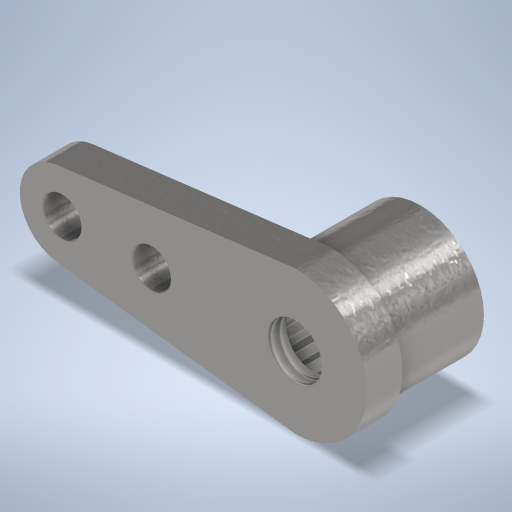
# Autodesk Inventor part: ara parca2
Saved by Autodesk Inventor 2023 (Build 270158000, 158)
## iProperties
Created: 2023-02-02
Part Number: ara parca2
Material: Generic
Document SubType Name: Sheet Metal
Designer: omuru
Density: 1 g/cm^3
Sheet Metal Rule: Default_mm
Appearance: Default
Author: omuru
Autodesk Inventor part; units mm, degrees
ref_plane "YZ Plane" through (0, 0, 0) normal (1, 0, 0) x (0, 1, 0)
ref_plane "XZ Plane" through (0, 0, 0) normal (0, 1, 0) x (-1, 0, 0)
ref_plane "XY Plane" through (0, 0, 0) normal (0, 0, 1) x (1, 0, 0)
sketch "Sketch1" plane through (0, 0, 0) normal (0, 0, 1) x (1, 0, 0)
  circle A0 centre (0, 0) radius 4
  circle A1 centre (0, 0) radius 3.5
  line L0 (0, 0) -> (-13, 0)
  line L1 (-13, 0) -> (-13, 0)
  circle A2 centre (-13, 0) radius 1.075
  line L2 (-13, 0) -> (-8, 0)
  circle A3 centre (-8, 0) radius 1.075
  arc A4 (-13.2917, 2.3513) -> (-13.2917, -2.3513) centre (-13, 0) ccw
  line L3 (0, 4) -> (-13.2917, 2.3513)
  line L4 (0, -4) -> (-13.2917, -2.3513)
  dimension "d0" = 8
  dimension "d1" = 7
  dimension "d5" = 2.15
  dimension "d7" = 2.15
  dimension "d31" = 8
  dimension "d33" = 5
  constraints: 10 end point, 6 coincident, 5 centre point, 4 point on circle, 2 point on line, 2 tangent, 1 horizontal
  measures "d0" diameter of A0
  measures "d1" diameter of A1
  measures "d5" diameter of A2
  measures "d7" diameter of A3
  measures "d31" distance of point (0, 0) L2.end
  measures "d33" distance of A3.centre L2.start
extrude "Extrusion1" add sketch "Sketch1" along normal mid plane 2 contours A0 L4 L3 | A0 L4 A4 L3
sketch "Sketch2" plane through (0, 0, -1) normal (0, 0, -1) x (-1, 0, 0)
  circle A0 centre (0, 0) radius 2.5
  circle A1 centre (0, 0) radius 4
  dimension "d11" = 5
  constraints: 2 centre point, 2 coincident
  measures "d11" diameter of A0
extrude "Extrusion2" add sketch "Sketch2" against normal blind 1
sketch "Sketch3" plane through (0, 0, 1) normal (0, 0, 1) x (1, 0, 0)
  circle A0 centre (0, 0) radius 3
  line L0 (0, 3) -> (0, 2.5)
  circle A1 centre (0, 0) radius 2.5 projected
  line L1 (-0.7461, 2.9057) -> (-0.6217, 2.4215)
  line L2 (-1.4453, 2.6289) -> (-1.2044, 2.1908)
  line L3 (-2.0536, 2.1869) -> (-1.7114, 1.8224)
  line L4 (-2.533, 1.6075) -> (-2.1108, 1.3396)
  line L5 (-2.8532, 0.9271) -> (-2.3776, 0.7725)
  line L6 (-2.9941, 0.1884) -> (-2.4951, 0.157)
  line L7 (-2.9469, -0.5621) -> (-2.4557, -0.4685)
  line L8 (-2.7145, -1.2773) -> (-2.2621, -1.0644)
  line L9 (-2.3115, -1.9123) -> (-1.9263, -1.5936)
  line L10 (-1.7634, -2.4271) -> (-1.4695, -2.0225)
  line L11 (-1.1044, -2.7893) -> (-0.9203, -2.3244)
  line L12 (-0.376, -2.9763) -> (-0.3133, -2.4803)
  line L13 (0.376, -2.9763) -> (0.3133, -2.4803)
  line L14 (1.1044, -2.7893) -> (0.9203, -2.3244)
  line L15 (1.7634, -2.4271) -> (1.4695, -2.0225)
  line L16 (2.3115, -1.9123) -> (1.9263, -1.5936)
  line L17 (2.7145, -1.2773) -> (2.2621, -1.0644)
  line L18 (2.9469, -0.5621) -> (2.4557, -0.4685)
  line L19 (2.9941, 0.1884) -> (2.4951, 0.157)
  line L20 (2.8532, 0.9271) -> (2.3776, 0.7725)
  line L21 (2.533, 1.6075) -> (2.1108, 1.3396)
  line L22 (2.0536, 2.1869) -> (1.7114, 1.8224)
  line L23 (1.4453, 2.6289) -> (1.2044, 2.1908)
  line L24 (0.7461, 2.9057) -> (0.6217, 2.4215)
  line L25 (-0.3133, 2.4803) -> (-0.7461, 2.9057)
  line L26 (-0.3133, 2.4803) -> (0, 3)
  line L27 (0, 3) -> (0.3133, 2.4803)
  line L28 (0.3133, 2.4803) -> (0.7461, 2.9057)
  circle A2 centre (0, 0) radius 2.5
  line L29 (-0.9203, 2.3244) -> (-0.7461, 2.9057)
  line L30 (-0.7461, 2.9057) -> (-0.3133, 2.4803)
  circle A3 centre (0, 0) radius 2.5
  line L31 (-1.4695, 2.0225) -> (-1.4453, 2.6289)
  line L32 (-1.4453, 2.6289) -> (-0.9203, 2.3244)
  circle A4 centre (0, 0) radius 2.5
  line L33 (-1.9263, 1.5936) -> (-2.0536, 2.1869)
  line L34 (-2.0536, 2.1869) -> (-1.4695, 2.0225)
  circle A5 centre (0, 0) radius 2.5
  line L35 (-2.2621, 1.0644) -> (-2.533, 1.6075)
  line L36 (-2.533, 1.6075) -> (-1.9263, 1.5936)
  circle A6 centre (0, 0) radius 2.5
  line L37 (-2.4557, 0.4685) -> (-2.8532, 0.9271)
  line L38 (-2.8532, 0.9271) -> (-2.2621, 1.0644)
  circle A7 centre (0, 0) radius 2.5
  line L39 (-2.4951, -0.157) -> (-2.9941, 0.1884)
  line L40 (-2.9941, 0.1884) -> (-2.4557, 0.4685)
  circle A8 centre (0, 0) radius 2.5
  line L41 (-2.3776, -0.7725) -> (-2.9469, -0.5621)
  line L42 (-2.9469, -0.5621) -> (-2.4951, -0.157)
  circle A9 centre (0, 0) radius 2.5
  line L43 (-2.1108, -1.3396) -> (-2.7145, -1.2773)
  line L44 (-2.7145, -1.2773) -> (-2.3776, -0.7725)
  circle A10 centre (0, 0) radius 2.5
  line L45 (-1.7114, -1.8224) -> (-2.3115, -1.9123)
  line L46 (-2.3115, -1.9123) -> (-2.1108, -1.3396)
  circle A11 centre (0, 0) radius 2.5
  line L47 (-1.2044, -2.1908) -> (-1.7634, -2.4271)
  line L48 (-1.7634, -2.4271) -> (-1.7114, -1.8224)
  circle A12 centre (0, 0) radius 2.5
  line L49 (-0.6217, -2.4215) -> (-1.1044, -2.7893)
  line L50 (-1.1044, -2.7893) -> (-1.2044, -2.1908)
  circle A13 centre (0, 0) radius 2.5
  line L51 (0, -2.5) -> (-0.376, -2.9763)
  line L52 (-0.376, -2.9763) -> (-0.6217, -2.4215)
  circle A14 centre (0, 0) radius 2.5
  line L53 (0.6217, -2.4215) -> (0.376, -2.9763)
  line L54 (0.376, -2.9763) -> (0, -2.5)
  circle A15 centre (0, 0) radius 2.5
  line L55 (1.2044, -2.1908) -> (1.1044, -2.7893)
  line L56 (1.1044, -2.7893) -> (0.6217, -2.4215)
  circle A16 centre (0, 0) radius 2.5
  line L57 (1.7114, -1.8224) -> (1.7634, -2.4271)
  line L58 (1.7634, -2.4271) -> (1.2044, -2.1908)
  circle A17 centre (0, 0) radius 2.5
  line L59 (2.1108, -1.3396) -> (2.3115, -1.9123)
  line L60 (2.3115, -1.9123) -> (1.7114, -1.8224)
  circle A18 centre (0, 0) radius 2.5
  line L61 (2.3776, -0.7725) -> (2.7145, -1.2773)
  line L62 (2.7145, -1.2773) -> (2.1108, -1.3396)
  circle A19 centre (0, 0) radius 2.5
  line L63 (2.4951, -0.157) -> (2.9469, -0.5621)
  line L64 (2.9469, -0.5621) -> (2.3776, -0.7725)
  circle A20 centre (0, 0) radius 2.5
  line L65 (2.4557, 0.4685) -> (2.9941, 0.1884)
  line L66 (2.9941, 0.1884) -> (2.4951, -0.157)
  circle A21 centre (0, 0) radius 2.5
  line L67 (2.2621, 1.0644) -> (2.8532, 0.9271)
  line L68 (2.8532, 0.9271) -> (2.4557, 0.4685)
  circle A22 centre (0, 0) radius 2.5
  line L69 (1.9263, 1.5936) -> (2.533, 1.6075)
  line L70 (2.533, 1.6075) -> (2.2621, 1.0644)
  circle A23 centre (0, 0) radius 2.5
  line L71 (1.4695, 2.0225) -> (2.0536, 2.1869)
  line L72 (2.0536, 2.1869) -> (1.9263, 1.5936)
  circle A24 centre (0, 0) radius 2.5
  line L73 (0.9203, 2.3244) -> (1.4453, 2.6289)
  line L74 (1.4453, 2.6289) -> (1.4695, 2.0225)
  circle A25 centre (0, 0) radius 2.5
  line L75 (0.3133, 2.4803) -> (0.7461, 2.9057)
  line L76 (0.7461, 2.9057) -> (0.9203, 2.3244)
  circle A26 centre (0, 0) radius 2.5
  circle A27 centre (0, 0) radius 3.5405
  dimension "d15" = 6
  dimension "d18" = 360
  dimension "d22" = 360
  constraints: 154 end point, 27 centre point, 3 coincident, 2 point on circle, 1 vertical, 257 other
  measures "d15" diameter of A0
extrude "Extrusion3" cut sketch "Sketch3" against normal blind 10 contours L66 A1 L19 | L19 A1 L65 | L64 A1 L18 | L18 A1 L63 | L68 A1 L20 | L20 A1 L67 | L62 A1 L17 | L17 A1 L61 | L70 A1 L21 | L21 A1 L69 | L60 A1 L16 | L16 A1 L59 | L72 A1 L22 | L22 A1 L71 | L58 A1 L15 | L15 A1 L57 | L74 A1 L23 | L23 A1 L73 | L56 A1 L14 | L14 A1 L55 | L76 A1 L24 | L24 A1 L28 | L54 A1 L13 | L13 A1 L53 | L27 A1 L0 | L0 A1 L26 | L52 A1 L12 | L12 A1 L51 | L25 A1 L1 | L1 A1 L29 | L50 A1 L11 | L11 A1 L49 | L32 A1 L2 | L2 A1 L31 | L48 A1 L10 | L10 A1 L47 | L34 A1 L3 | L3 A1 L33 | L46 A1 L9 | L9 A1 L45 | L36 A1 L4 | L4 A1 L35 | L44 A1 L8 | L8 A1 L43 | L38 A1 L5 | L5 A1 L37 | L42 A1 L7 | L7 A1 L41 | L40 A1 L6 | L6 A1 L39
sketch "Sketch4" plane through (0, 0, 1) normal (0, 0, 1) x (1, 0, 0)
  circle A0 centre (0, 0) radius 3.5
  circle A1 centre (0, 0) radius 1.5
  dimension "d35" = 3
  constraints: 2 centre point, 2 coincident
  measures "d35" diameter of A1
extrude "Extrusion4" add sketch "Sketch3" against normal blind 7 contours A0 L63 L66 | L65 L68 A0 | A0 L61 L64 | L67 L70 A0 | A0 L59 L62 | L69 L72 A0 | A0 L57 L60 | L71 L74 A0 | A0 L55 L58 | L73 L76 A0 | A0 L53 L56 | L28 L27 A0 | A0 L51 L54 | L26 L25 A0 | A0 L49 L52 | L29 L32 A0 | A0 L47 L50 | L31 L34 A0 | A0 L45 L48 | L33 L36 A0 | A0 L43 L46 | L35 L38 A0 | A0 L41 L44 | L37 L40 A0 | A0 L39 L42 | A27
extrude "Extrusion5" add sketch "Sketch4" against normal blind 1
fillet "Fillet3" radius 0.05 4 edges at (-2.4557, 0.4685, -0.5) (-2.4557, 0.4685, -3.5) (-2.9941, 0.1884, -0.5) (-2.9941, 0.1884, -3.5)
pattern_circular "Circular Pattern2" count 25 over 360 about axis through (0, 0, 1) along (0, 0, -1) of "Fillet3"
thread "Thread1" size "M3x0.5" class "6H" standard "ANSI Metric M Profile" full length
equation "\"BendRadius\" = Thickness"
equation "\"BendReliefWidth\" = Thickness"
equation "\"BendReliefDepth\" = 0.5 * Thickness"
equation "\"CornerReliefSize\" = 4 * Thickness"
equation "\"MinimumRemnant\" = 2 * Thickness"
equation "\"TransitionRadius\" = BendRadius"
equation "\"JacobiRadiusSize\" = BendRadius"
equation "\"GapSize\" = Thickness"
equation "\"Thickness\" = 0.5"
body "Solid1"
